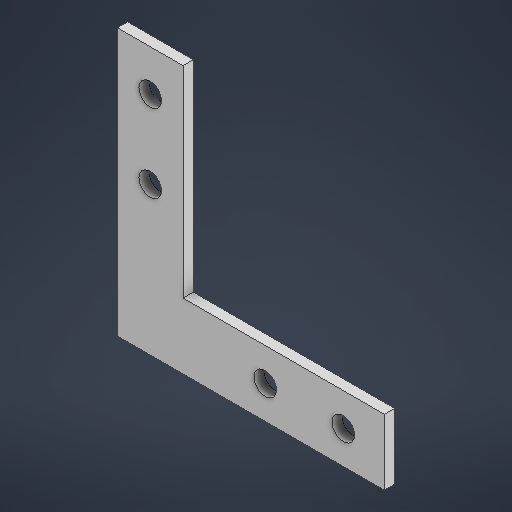
# Autodesk Inventor part: L型
Saved by Autodesk Inventor 2025 (Build 290162000, 162)
## iProperties
Created: 2025-06-23
Part Number: L型
Material: 常规
Document SubType Name: Modeling
Designer: HZD
Density: 1 g/cm^3
Appearance: 默认
Author: HZD
Autodesk Inventor part; units mm, degrees
ref_plane "YZ Plane" through (0, 0, 0) normal (1, 0, 0) x (0, 1, 0)
ref_plane "XZ Plane" through (0, 0, 0) normal (0, 1, 0) x (-1, 0, 0)
ref_plane "XY Plane" through (0, 0, 0) normal (0, 0, 1) x (1, 0, 0)
sketch "草图1" plane through (0, 0, 0) normal (0, 0, 1) x (1, 0, 0)
  line L0 (0, 0) -> (-16, 0)
  line L1 (-16, 0) -> (-16, 65)
  line L2 (-16, 65) -> (0, 65)
  line L3 (0, 65) -> (0, 0)
  line L4 (-16, 16) -> (49, 16)
  line L5 (49, 16) -> (49, 0)
  line L6 (49, 0) -> (-16, 0)
  line L7 (-16, 0) -> (-16, 16)
  line L8 (-8, 65) -> (-8, 0)
  line L9 (-16, 8) -> (49, 8)
  circle A0 centre (-8, 55) radius 2.75
  circle A1 centre (-8, 36) radius 2.75
  circle A2 centre (39, 8) radius 2.75
  circle A3 centre (20, 8) radius 2.75
  point P0 (0, 16)
  dimension "d0" = 65
  dimension "d1" = 65
  dimension "d2" = 16
  dimension "d3" = 16
  dimension "d4" = 5.5
  dimension "d5" = 5.5
  dimension "d6" = 19
  dimension "d7" = 10
  dimension "d8" = 5.5
  dimension "d9" = 5.5
  dimension "d10" = 19
  dimension "d11" = 10
  constraints: 20 end point, 6 point on line, 4 centre point, 4 parallel, 3 midpoint, 3 perpendicular, 2 horizontal
  measures "d0" distance between parallel lines of L1 L5
  measures "d1" distance between parallel lines of L2 L0
  measures "d2" distance of L1.end L2.end
  measures "d3" distance of L4.end L5.end
  measures "d4" diameter of A0
  measures "d5" diameter of A1
  measures "d6" distance of A1.centre A0.centre
  measures "d7" distance from line of A0.centre L2
  measures "d8" diameter of A2
  measures "d9" diameter of A3
  measures "d10" distance of A3.centre A2.centre
  measures "d11" distance from line of A2.centre L5
extrude "拉伸1" add sketch "草图1" along normal blind 2.5 contours L0 L8 L9 L3 | L3 L9 A3 A2 L5 L6 | L0 L1 L9 L8 | L9 L8 L4 L3 | L3 L4 L5 L9 A2 A3 | L9 L1 L4 L8 | L4 L8 A1 A0 L2 L3 | L4 L1 L2 L8 A0 A1
